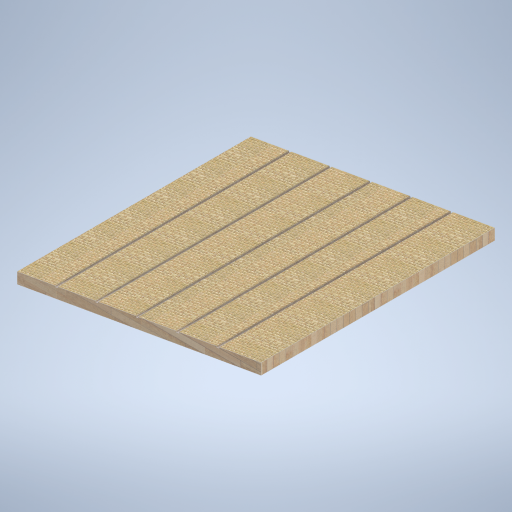
# Autodesk Inventor part: eave_panel_side_
Saved by Autodesk Inventor 2024.2 (Build 282272000, 272)
## iProperties
Created: 2024-05-24
Part Number: eave_panel_side_
Material: Wood (Maple)
Document SubType Name: Modeling
Designer: LOSTER_1
Density: 0.67 g/cm^3
Appearance: Natural Maple - Glossy Dark Tint
Author: LOSTER_1
Autodesk Inventor part; units mm, degrees
ref_plane "YZ Plane" through (0, 0, 0) normal (1, 0, 0) x (0, 1, 0)
ref_plane "XZ Plane" through (0, 0, 0) normal (0, 1, 0) x (-1, 0, 0)
ref_plane "XY Plane" through (0, 0, 0) normal (0, 0, 1) x (1, 0, 0)
sketch "Sketch1" plane through (0, 0, 0) normal (1, 0, 0) x (0, 1, 0)
  line L0 (-50, 1054) -> (50, 1054)
  line L1 (50, 1054) -> (50, -1054)
  line L2 (50, -1054) -> (-50, -1054)
  line L3 (-50, -1054) -> (-50, 1054)
  line L4 (-50, 1054) -> (50, -1054) construction
  line L5 (50, 1054) -> (-50, -1054) construction
  point P0 (0, 0)
  dimension "d0" = 100
  dimension "d1" = 2108
  constraints: 12 end point, 2 midpoint, 2 parallel, 1 horizontal, 1 perpendicular
  measures "d0" distance of L1.end L2.end
  measures "d1" distance of L0.end L1.end
ref_plane "Work Plane2" through (-2200, 50, 1054) normal (-1, 0, 0) x (0, 0, -1)
ref_plane "Work Plane1" through (0, 50, 1054) normal (-1, 0, 0) x (0, 0, -1)
sketch "Sketch2" plane through (-2200, 50, 1054) normal (-1, 0, 0) x (0, 0, -1)
  line L0 (0, 0) -> (2108, 0) projected
  line L1 (2108, 0) -> (2108, 100) projected
  line L2 (0, 100) -> (0, 0) projected
  point P0 (1054, 50)
ref_plane "Work Plane3" through (0, 50, -1054) normal (0, 0, -1) x (0, -1, 0)
sketch "Sketch3" plane through (0, 50, -1054) normal (0, 0, -1) x (0, -1, 0)
  line L0 (0, 0) -> (100, 0) projected
  line L1 (0, 2200) -> (100, 2200) projected
  line L2 (0, 0) -> (387.9194, 2200)
  line L3 (0, 0) -> (2233.9385, 0) construction
  line L4 (100, 0) -> (487.9194, 2200)
  line L5 (100, 0) -> (2333.9385, 0) construction
  line L6 (487.9194, 2200) -> (387.9194, 2200)
  line L7 (0, 0) -> (100, 0)
  point P0 (50, 0)
  dimension "d3" = 80
  dimension "d4" = 80
  constraints: 12 end point, 3 horizontal, 2 equal length, 1 parallel
  measures "d3" angle of L3 L2
  measures "d4" angle of L5 L4
extrude "Extrusion1" add sketch "Sketch3" against normal blind 2108
sketch "Sketch4" plane through (0, 50, 1054) normal (0, 0, 1) x (1, 0, 0)
  line L0 (0, 0) -> (-2200, -387.9194) projected
  line L1 (-2200, -387.9194) -> (-1855.3173, -327.1425)
  line L2 (-1855.3173, -327.1425) -> (-1855.3173, -337.4554)
  line L3 (-1855.3173, -337.4554) -> (-1835.3641, -333.9371)
  line L4 (-1835.3641, -333.9371) -> (-1835.3641, -323.6242)
  line L5 (-1835.3641, -323.6242) -> (-1490.6814, -262.8474)
  line L6 (-1490.6814, -262.8474) -> (-1490.6814, -273.1602)
  line L7 (-1490.6814, -273.1602) -> (-1471.2413, -269.7324)
  line L8 (-1471.2413, -269.7324) -> (-1471.2413, -259.4195)
  line L9 (-1471.2413, -259.4195) -> (-1126.5586, -198.6427)
  line L10 (-1126.5586, -198.6427) -> (-1126.5586, -208.9555)
  line L11 (-1126.5586, -208.9555) -> (-1107.1904, -205.5404)
  line L12 (-1107.1904, -205.5404) -> (-1107.1904, -195.2275)
  line L13 (-1107.1904, -195.2275) -> (-762.5076, -134.4507)
  line L14 (-762.5076, -134.4507) -> (-762.5076, -144.7635)
  line L15 (-762.5076, -144.7635) -> (-742.5762, -141.2491)
  line L16 (-742.5762, -141.2491) -> (-742.5762, -130.9362)
  line L17 (-742.5762, -130.9362) -> (-397.8935, -70.1594)
  line L18 (-397.8935, -70.1594) -> (-397.8935, -80.4722)
  line L19 (-397.8935, -80.4722) -> (-377.71, -76.9133)
  line L20 (-377.71, -76.9133) -> (-377.71, -66.6005)
  line L21 (-377.71, -66.6005) -> (0, 0)
  line L22 (-377.71, -66.6005) -> (-1855.3173, -327.1425)
  point P0 (0, -50)
  dimension "d7" = 350
  dimension "d8" = 350
  dimension "d9" = 350
  dimension "d10" = 350
  dimension "d11" = 350
  constraints: 44 end point, 9 parallel, 7 point on line, 1 coincident, 1 vertical, 12 other
  measures "d7" distance of L1.start L1.end
  measures "d8" distance of L4.end L5.end
  measures "d9" distance of L8.end L9.end
  measures "d10" distance of L12.end L13.end
  measures "d11" distance of L16.end L17.end
extrude "Extrusion2" cut sketch "Sketch4" against normal through all
body "Solid1"
